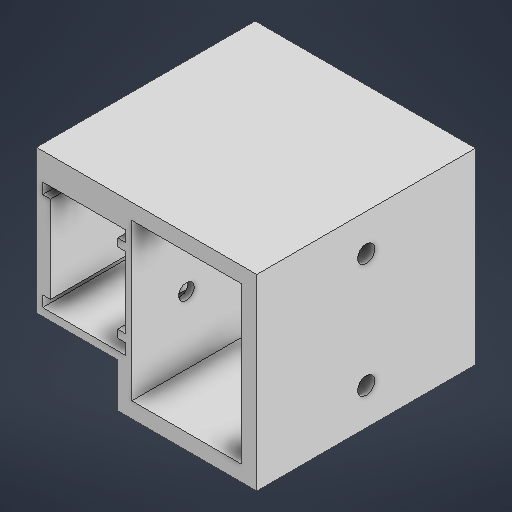
# Autodesk Inventor part: baseGuias
Saved by Autodesk Inventor 2025.3 (Build 293356000, 356)
## iProperties
Created: 2025-10-14
Part Number: baseGuias
Material: Genérico
Document SubType Name: Modeling
Designer: Jonathan Galarza
Density: 1 g/cm^3
Appearance: Valor por defecto
Author: Jonathan Galarza
Autodesk Inventor part; units mm, degrees
ref_plane "YZ Plane" through (0, 0, 0) normal (1, 0, 0) x (0, 1, 0)
ref_plane "XZ Plane" through (0, 0, 0) normal (0, 1, 0) x (-1, 0, 0)
ref_plane "XY Plane" through (0, 0, 0) normal (0, 0, 1) x (1, 0, 0)
sketch "Boceto1" plane through (0, 0, 0) normal (0, 1, 0) x (-1, 0, 0)
  line L0 (-30, -35) -> (30, -35)
  line L1 (30, -35) -> (30, 35)
  line L2 (30, 35) -> (-30, 35)
  line L3 (-30, 35) -> (-30, -35)
  line L4 (-30, -35) -> (30, 35) construction
  line L5 (30, -35) -> (-30, 35) construction
  point P0 (0, 0)
  dimension "d0" = 60
  dimension "d1" = 70
  constraints: 12 end point, 2 midpoint, 2 parallel, 1 horizontal, 1 perpendicular
  measures "d0" distance of L2.end L1.end
  measures "d1" distance of L1.end L0.end
extrude "Extrusión1" add sketch "Boceto1" along normal blind 5
sketch "Boceto2" plane through (0, 5, 0) normal (0, 1, 0) x (1, 0, 0)
  line L0 (-30, 35) -> (-30, -35) projected
  line L1 (-30, 0) -> (7.5, 0)
  line L2 (30, -35) -> (30, 35) projected
  line L3 (30, 0) -> (18, 0)
  circle A0 centre (18, 0) radius 5
  circle A1 centre (18, 25) radius 5
  circle A2 centre (18, -25) radius 5
  point P0 (0, 0)
  point P1 (24, 0)
  dimension "d4" = 37.5
  dimension "d5" = 12
  dimension "d6" = 10
  dimension "d8" = 10
  dimension "d9" = 25
  constraints: 4 end point, 3 centre point, 3 midpoint, 2 horizontal, 1 coincident, 1 symmetric about line, 1 other
  measures "d4" distance of L1.start L1.end
  measures "d5" distance of L3.start L3.end
  measures "d6" diameter of A0
  measures "d8" diameter of A1
  measures "d9" vertical distance of point (24, 0) A1.centre
extrude "Extrusión2" cut sketch "Boceto2" against normal blind 5
sketch "Boceto3" plane through (0, 0, 0) normal (0, -1, 0) x (1, 0, 0)
  line L0 (-30, 35) -> (30, 35) projected
  line L1 (-30, 35) -> (-58.5, 35)
  line L2 (-58.5, 35) -> (-58.5, -35)
  line L3 (-58.5, -35) -> (-30, -35)
  line L4 (-30, -35) -> (-30, 35)
  point P0 (0, 0)
  dimension "d12" = 28.5
  dimension "d13" = 70
  constraints: 8 end point, 2 parallel, 1 horizontal, 1 perpendicular
  measures "d12" distance of L3.end L2.end
  measures "d13" distance of L2.end L1.end
extrude "Extrusión3" add sketch "Boceto3" along normal blind 3.608 and the other way blind 5
sketch "Boceto4" plane through (0, -3.608, 0) normal (0, -1, 0) x (1, 0, 0)
  line L0 (-30, 35) -> (-58.5, 35) projected
  line L1 (-30, 35) -> (-32, 35)
  line L2 (-32, 35) -> (-32, -35)
  line L3 (-32, -35) -> (-30, -35)
  line L4 (-30, -35) -> (-30, 35)
  point P0 (0, 0)
  dimension "d18" = 2
  dimension "d19" = 70
  constraints: 8 end point, 2 parallel, 1 horizontal, 1 perpendicular
  measures "d18" distance of L3.end L2.end
  measures "d19" distance of L2.end L1.end
extrude "Extrusión4" add sketch "Boceto4" along normal blind 3.5
sketch "Boceto5" plane through (-30, 0, 35) normal (1, 0, 0) x (0, 0, -1)
  line L0 (70, -7.108) -> (0, -7.108) projected
  line L1 (70, -7.108) -> (0, -7.108)
  line L2 (0, -7.108) -> (0, -9.608)
  line L3 (0, -9.608) -> (70, -9.608)
  line L4 (70, -9.608) -> (70, -7.108)
  point P0 (35, 0)
  point P1 (0, -7.108)
  dimension "d22" = 70
  dimension "d23" = 2.5
  constraints: 8 end point, 2 parallel, 1 horizontal, 1 perpendicular
  measures "d22" distance of L3.end L2.end
  measures "d23" distance of L2.end L1.end
extrude "Extrusión5" add sketch "Boceto5" against normal blind 4.5
sketch "Boceto6" plane through (0, 5, 0) normal (0, 1, 0) x (1, 0, 0)
  line L0 (-58.5, 35) -> (-58.5, -35) projected
  line L1 (-58.5, 35) -> (-60.5, 35)
  line L2 (-60.5, 35) -> (-60.5, -35)
  line L3 (-60.5, -35) -> (-58.5, -35)
  line L4 (-58.5, -35) -> (-58.5, 35)
  point P0 (0, 0)
  dimension "d26" = 2
  dimension "d27" = 70
  constraints: 8 end point, 2 parallel, 1 horizontal, 1 perpendicular
  measures "d26" distance of L3.end L2.end
  measures "d27" distance of L2.end L1.end
extrude "Extrusión6" add sketch "Boceto6" against normal blind 12.358
sketch "Boceto8" plane through (-60.5, 5, -35) normal (-1, 0, 0) x (0, 0, 1)
  line L0 (70, -8.608) -> (70, -12.108) projected
  line L1 (70, -12.108) -> (0, -12.108)
  line L2 (0, -12.108) -> (0, -39.893)
  line L3 (0, -39.893) -> (70, -39.893)
  line L4 (70, -39.893) -> (70, -12.108)
  point P0 (35, -5)
  dimension "d34" = 70
  dimension "d35" = 27.785
  constraints: 8 end point, 2 parallel, 1 horizontal, 1 perpendicular
  measures "d34" distance of L3.end L2.end
  measures "d35" distance of L2.end L1.end
extrude "Extrusión8" add sketch "Boceto8" against normal blind 4.5
sketch "Boceto9" plane through (-60.5, -34.893, -35) normal (0, -1, 0) x (1, 0, 0)
  line L0 (0, 0) -> (4.5, 0) projected
  line L1 (0, 0) -> (2, 0)
  line L2 (2, 0) -> (2, 70)
  line L3 (2, 70) -> (0, 70)
  line L4 (0, 70) -> (0, 0)
  point P0 (60.5, 35)
  point P1 (2, 0)
  dimension "d38" = 2
  dimension "d39" = 70
  constraints: 8 end point, 2 parallel, 1 horizontal, 1 perpendicular
  measures "d38" distance of L3.end L2.end
  measures "d39" distance of L2.end L1.end
extrude "Extrusión9" add sketch "Boceto9" along normal blind 3.5
sketch "Boceto15" plane through (-60.5, -38.393, -35) normal (0, -1, 0) x (1, 0, 0)
  line L0 (0, 0) -> (30.5, 0)
  line L1 (30.5, 0) -> (30.5, 70)
  line L2 (30.5, 70) -> (0, 70)
  line L3 (0, 70) -> (0, 0)
  point P0 (60.5, 35)
  dimension "d60" = 30.5
  dimension "d61" = 70
  constraints: 8 end point, 2 parallel, 1 horizontal, 1 perpendicular, 1 point on line
  measures "d60" distance of L2.end L1.end
  measures "d61" distance of L1.end L0.end
extrude "Extrusión15" add sketch "Boceto15" along normal blind 2.5
sketch "Boceto16" plane through (-60.5, -38.393, -35) normal (0, 1, 0) x (1, 0, 0)
  line L0 (30.5, 0) -> (30.5, -70) projected
  line L1 (30.5, 0) -> (28.5, 0)
  line L2 (28.5, 0) -> (28.5, -70)
  line L3 (28.5, -70) -> (30.5, -70)
  line L4 (30.5, -70) -> (30.5, 0)
  point P0 (60.5, -35)
  dimension "d64" = 2
  dimension "d65" = 70
  constraints: 8 end point, 2 parallel, 1 horizontal, 1 perpendicular
  measures "d64" distance of L3.end L2.end
  measures "d65" distance of L2.end L1.end
extrude "Extrusión16" add sketch "Boceto16" along normal blind 3.5
sketch "Boceto17" plane through (-30, -40.893, 35) normal (1, 0, 0) x (0, 0, -1)
  line L0 (70, 6) -> (70, 2.5) projected
  line L1 (70, 6) -> (0, 6)
  line L2 (0, 6) -> (0, 8.5)
  line L3 (0, 8.5) -> (70, 8.5)
  line L4 (70, 8.5) -> (70, 6)
  point P0 (35, 40.893)
  dimension "d68" = 70
  dimension "d69" = 2.5
  constraints: 8 end point, 2 parallel, 1 horizontal, 1 perpendicular
  measures "d68" distance of L2.end L3.end
  measures "d69" distance of L1.end L2.end
extrude "Extrusión17" add sketch "Boceto17" against normal blind 4.5
sketch "Boceto18" plane through (-30, -40.893, 35) normal (1, 0, 0) x (0, 0, -1)
  line L0 (70, 8.5) -> (70, 6) projected
  line L1 (0, 45.893) -> (0, 0) projected
  line L2 (70, 8.5) -> (0, 8.5)
  line L3 (0, 8.5) -> (0, 32.8457)
  line L4 (0, 32.8457) -> (70, 32.8457)
  line L5 (70, 32.8457) -> (70, 8.5)
  point P0 (35, 40.893)
  point P1 (0, 8.5)
  constraints: 8 end point, 2 parallel, 1 horizontal, 1 perpendicular, 1 point on line
extrude "Extrusión18" add sketch "Boceto18" against normal blind 2
sketch "Boceto19" plane through (-30, 0, 35) normal (1, 0, 0) x (0, 0, -1)
  line L0 (0, -40.893) -> (70, -40.893) projected
  line L1 (70, -40.893) -> (0, 0) construction
  line L2 (0, 5) -> (0, -40.893) projected
  line L3 (0, -40.893) -> (70, 0) construction
  line L4 (70, 5) -> (70, -40.893) projected
  circle A0 centre (35, -20.4465) radius 4.75
  point P0 (35, 0)
  dimension "d74" = 9.5
  constraints: 4 end point, 2 point on line, 1 centre point, 1 midpoint
  measures "d74" diameter of A0
extrude "Extrusión19" cut sketch "Boceto19" against normal blind 5
sketch "Boceto20" plane through (-60.5, 5, -35) normal (-1, 0, 0) x (0, 0, 1)
  circle A0 centre (35, -25.4465) radius 4.75 projected
  line L0 (70, -5) -> (70, -45.893) projected
  line L1 (0, -45.893) -> (70, -45.893) projected
  line L2 (0, -5) -> (0, -45.893) projected
  line L3 (0, -5) -> (70, -5) projected
  circle A1 centre (35, -25.4465) radius 2.5
  point P0 (35, -5)
  dimension "d77" = 5
  constraints: 1 centre point, 1 coincident
  measures "d77" diameter of A1
extrude "Extrusión20" add sketch "Boceto20" against normal blind 7 contours A1
sketch "Boceto21" plane through (-30, 0, 35) normal (1, 0, 0) x (0, 0, -1)
  circle A0 centre (35, -20.4465) radius 4.75 projected
  circle A1 centre (35, -20.4465) radius 2.5 projected
  line L0 (35, -20.4465) -> (35, -28.4465) construction
  line L1 (52.5, -28.4465) -> (17.5, -28.4465) construction
  circle A2 centre (52.5, -28.4465) radius 2.5
  circle A3 centre (17.5, -28.4465) radius 2.5
  point P0 (35, 0)
  dimension "d80" = 8
  dimension "d81" = 35
  dimension "d82" = 5
  dimension "d83" = 5
  constraints: 4 end point, 2 centre point, 2 coincident, 1 horizontal, 1 midpoint, 1 vertical
  measures "d80" distance of L0.end L0.start
  measures "d81" distance of L1.start L1.end
  measures "d82" diameter of A2
  measures "d83" diameter of A3
extrude "Extrusión21" cut sketch "Boceto21" against normal blind 5 contours A2 | A3
sketch "Boceto22" plane through (30, 0, 35) normal (1, 0, 0) x (0, 0, -1)
  line L0 (100.391, -19.241) -> (-19.599, -19.241)
  line L1 (-19.599, -19.241) -> (-19.599, 22.649)
  line L2 (-19.599, 22.649) -> (100.391, 22.649)
  line L3 (100.391, 22.649) -> (100.391, -19.241)
  point P0 (35, 0)
  constraints: 8 end point, 2 parallel, 1 horizontal, 1 perpendicular
extrude "Extrusión22" cut sketch "Boceto22" against normal blind 25
sketch "Boceto23" plane through (0, 5, 0) normal (0, 1, 0) x (1, 0, 0)
  line L0 (-60.5, -35) -> (5, -35) projected
  line L1 (5, -35) -> (10, -35)
  line L2 (10, -35) -> (10, 35)
  line L3 (10, 35) -> (5, 35)
  line L4 (5, 35) -> (5, -35)
  point P0 (0, 0)
  dimension "d88" = 5
  dimension "d89" = 70
  constraints: 8 end point, 2 parallel, 1 horizontal, 1 perpendicular
  measures "d88" distance of L3.end L2.end
  measures "d89" distance of L2.end L1.end
extrude "Extrusión23" add sketch "Boceto23" against normal blind 60
sketch "Boceto24" plane through (10, 5, 35) normal (1, 0, 0) x (0, 0, -1)
  line L0 (0, -60) -> (70, -60) projected
  line L1 (70, -60) -> (0, -60)
  line L2 (0, -60) -> (0, -55)
  line L3 (0, -55) -> (70, -55)
  line L4 (70, -55) -> (70, -60)
  point P0 (35, -5)
  dimension "d92" = 70
  dimension "d93" = 5
  constraints: 8 end point, 2 parallel, 1 horizontal, 1 perpendicular
  measures "d92" distance of L2.end L3.end
  measures "d93" distance of L1.end L2.end
extrude "Extrusión24" add sketch "Boceto24" against normal blind 40
sketch "Boceto25" plane through (-60.5, -40.893, -35) normal (0, -1, 0) x (1, 0, 0)
  line L0 (0, 0) -> (30.5, 0) projected
  line L1 (26, 70) -> (26, 0) projected
  line L2 (30.5, 0) -> (26, 0)
  line L3 (26, 0) -> (26, 70)
  line L4 (26, 70) -> (30.5, 70)
  line L5 (30.5, 70) -> (30.5, 0)
  point P0 (60.5, 35)
  dimension "d96" = 4.5
  dimension "d97" = 70
  constraints: 8 end point, 2 parallel, 1 horizontal, 1 perpendicular
  measures "d96" distance of L1.start L4.end
  measures "d97" distance of L2.end L1.start
extrude "Extrusión25" add sketch "Boceto25" along normal blind 14.107
sketch "Boceto26" plane through (10, 5, 35) normal (1, 0, 0) x (0, 0, -1)
  line L0 (70, -60) -> (0, -60) projected
  line L1 (70, 0) -> (70, -45.893) projected
  line L2 (0, -60) -> (70, 0) construction
  line L3 (0, 0) -> (70, 0) projected
  line L4 (0, 0) -> (70, -60) construction
  line L5 (35, -48.25) -> (35, -11.75) construction
  line L6 (70, -8.608) -> (0, -8.608) projected
  circle A0 centre (35, -48.25) radius 2.75
  circle A1 centre (35, -11.75) radius 2.75
  point P0 (35, -5)
  point P1 (35, -30)
  point P2 (35, -30)
  dimension "d103" = 36.5
  dimension "d104" = 5.5
  dimension "d105" = 5.5
  constraints: 6 end point, 3 midpoint, 2 centre point, 2 coincident, 1 perpendicular
  measures "d103" distance of L5.start L5.end
  measures "d104" diameter of A0
  measures "d105" diameter of A1
extrude "Extrusión26" cut sketch "Boceto26" against normal blind 14.107
equation "\"d84\" = d83"
